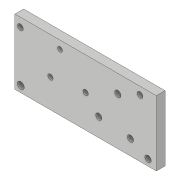
# Autodesk Inventor part: rectanglar
Saved by Autodesk Inventor 2019 (Build 230136000, 136)
## iProperties
Created: 2019-10-13
Part Number: rectanglar
Material: Generic
Document SubType Name: Sheet Metal
Designer: DELL PC
Density: 1 g/cm^3
Sheet Metal Rule: Default_mm
Appearance: Default
Author: DELL PC
Autodesk Inventor part; units mm, degrees
ref_plane "YZ Plane" through (0, 0, 0) normal (1, 0, 0) x (0, 1, 0)
ref_plane "XZ Plane" through (0, 0, 0) normal (0, 1, 0) x (-1, 0, 0)
ref_plane "XY Plane" through (0, 0, 0) normal (0, 0, 1) x (1, 0, 0)
sketch "Sketch1" plane through (0, 0, 0) normal (0, 0, 1) x (1, 0, 0)
  line L0 (32.5, -15) -> (-32.5, -15)
  line L1 (-32.5, -15) -> (-32.5, 15)
  line L2 (-32.5, 15) -> (32.5, 15)
  line L3 (32.5, 15) -> (32.5, -15)
  line L4 (32.5, -15) -> (-32.5, 15) construction
  line L5 (-32.5, -15) -> (32.5, 15) construction
  circle A0 centre (0, 0) radius 1.25
  circle A1 centre (-30, 11) radius 1.3364
  circle A2 centre (25, 11.5385) radius 1.3533
  circle A3 centre (31.3333, -14.4615) radius 1.3333
  circle A4 centre (-30, -15) radius 1.3333
  dimension "d0" = 30
  dimension "d1" = 65
  dimension "d2" = 2.5
  dimension "d3" = 26
  dimension "d4" = 26
  dimension "d5" = 55
  dimension "d6" = 25
  dimension "d7" = 15
  measures "d0" distance of L0.end L1.end
  measures "d1" distance of L1.end L2.end
  measures "d2" diameter of A0
  measures "d3" distance of A4.centre A1.centre
  measures "d4" vertical distance of A3.centre A2.centre
  measures "d5" horizontal distance of A2.centre A1.centre
  measures "d6" horizontal distance of A2.centre point (0, 0)
  measures "d7" vertical distance of point (0, 0) A4.centre
extrude "Plate1" add sketch "Sketch1" along normal blind 4 contours L0 A3 L3 | L0 A4 L1 L2 L3 A3 | L0 A4 picked at (30.9112, -14.2924) picked at (-29.6065, -14.7935)
sketch "Sketch2" plane through (0, 0, 4) normal (0, 0, 1) x (1, 0, 0)
  circle A0 centre (-29.8197, -12.1072) radius 1.6051
  circle A1 centre (28.6987, -12.1072) radius 1.4574
  point P0 (0, 0)
  constraints: 2 centre point
extrude "Extrusion1" cut sketch "Sketch2" against normal blind 5
sketch "Sketch3" plane through (0, 0, 4) normal (0, 0, 1) x (1, 0, 0)
  circle A0 centre (-27.5776, 6.8384) radius 0.7927
  circle A1 centre (-28.3703, -3.8115) radius 0.8238
  circle A2 centre (-16.143, -1.9058) radius 1.2074
  circle A3 centre (-11.7709, 11.3225) radius 1.1266
  circle A4 centre (6.0536, -6.6141) radius 1.4269
  circle A5 centre (14.7977, 6.8384) radius 1.466
  circle A6 centre (20.6272, -8.041) radius 1.4486
  point P0 (0, 0)
  constraints: 7 centre point
extrude "Extrusion2" cut sketch "Sketch3" against normal blind 5 contours A2 | A3 | A4 | A5 | A6
equation "\"d8\" = Thickness"
equation "\"BendRadius\" = Thickness"
equation "\"BendReliefWidth\" = Thickness"
equation "\"BendReliefDepth\" = 0.5 * Thickness"
equation "\"CornerReliefSize\" = 4 * Thickness"
equation "\"MinimumRemnant\" = 2 * Thickness"
equation "\"TransitionRadius\" = BendRadius"
equation "\"JacobiRadiusSize\" = BendRadius"
equation "\"GapSize\" = Thickness"
equation "\"Thickness\" = 4"
body "Solid1"
